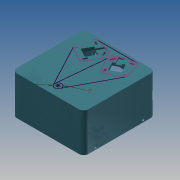
# Autodesk Inventor part: bottom plate box
Saved by Autodesk Inventor 2013 (Build 170138000, 138)
## iProperties
Created: 2017-03-31
Part Number: bottom plate box
Material: Generic
Document SubType Name: Modeling
Designer: employee
Density: 1 g/cm^3
Author: employee
Autodesk Inventor part; units mm, degrees
ref_plane "YZ Plane" through (0, 0, 0) normal (1, 0, 0) x (0, 1, 0)
ref_plane "XZ Plane" through (0, 0, 0) normal (0, 1, 0) x (-1, 0, 0)
sketch "Sketch1" plane through (0, 0, 0) normal (0, 0, 1) x (1, 0, 0)
  circle A0 centre (0, 0) radius 99 construction
  line L0 (0, 103.3586) -> (36.9795, 123.2713) construction
  line L1 (36.9795, 123.2713) -> (56.8922, 86.2918) construction
  line L2 (56.8922, 86.2918) -> (19.9127, 66.3791) construction
  line L3 (19.9127, 66.3791) -> (0, 103.3586) construction
  line L4 (19.9127, 66.3791) -> (0, 0) construction
  line L5 (34.7446, 115.8211) -> (7.4502, 101.1237) construction
  line L6 (7.4502, 101.1237) -> (22.1476, 73.8293) construction
  line L7 (22.1476, 73.8293) -> (49.442, 88.5267) construction
  line L8 (49.442, 88.5267) -> (34.7446, 115.8211) construction
  line L9 (45.2305, 125.1977) -> (56.1863, 84.6519) construction
  line L10 (56.1863, 84.6519) -> (15.6404, 73.696) construction
  line L11 (15.6404, 73.696) -> (4.6846, 114.2419) construction
  line L12 (30.4355, 99.4469) -> (28.9722, 94.6658) construction
  line L13 (0, 103.3586) -> (6.6568, 106.9431)
  line L14 (6.6568, 106.9431) -> (4.6846, 114.2419)
  line L15 (4.6846, 114.2419) -> (45.2305, 125.1977)
  line L16 (45.2305, 125.1977) -> (55.8891, 85.7517)
  line L17 (55.8891, 85.7517) -> (19.9127, 66.3791)
  line L18 (19.9127, 66.3791) -> (0, 103.3586)
  circle A1 centre (49.442, 88.5267) radius 1.75
  circle A2 centre (22.1476, 73.8293) radius 1.75
  circle A3 centre (7.4502, 101.1237) radius 1.75
  circle A4 centre (34.7446, 115.8211) radius 1.75
  line L19 (11.4289, 110.367) -> (41.3556, 118.4535) construction
  line L20 (41.3556, 118.4535) -> (49.442, 88.5267) construction
  line L21 (49.442, 88.5267) -> (19.5153, 80.4403) construction
  line L22 (19.5153, 80.4403) -> (11.4289, 110.367) construction
  circle A5 centre (19.5153, 80.4403) radius 1.75
  circle A6 centre (11.4289, 110.367) radius 1.75
  circle A7 centre (41.3556, 118.4535) radius 1.75
  point P0 (28.4461, 94.8252)
  point P1 (30.4355, 99.4469)
  dimension "d0" = 198
  dimension "d2" = 42
  dimension "d3" = 31
  dimension "d4" = 5.5
  dimension "d5" = 5.5
  dimension "d6" = 5
  dimension "d7" = 3.5
  dimension "d8" = 5.5
  dimension "d9" = 5.5
  constraints: 46 end point, 8 centre point, 8 coincident, 6 equal radius, 6 point on line, 3 collinear, 2 equal length, 2 point on circle, 1 parallel, 1 perpendicular, 1 vertical alignment, 28 other
  measures "d0" diameter of A0
  measures "d2" distance between parallel lines of L1 L3
  measures "d3" distance between parallel lines of L6 L8
  measures "d4" distance from line of L10 L7.end
  measures "d5" distance from line of L9 L7.end
  measures "d6" distance of L12.start L12.end
  measures "d7" diameter of A3
  measures "d8" distance between parallel lines of L22 L11
  measures "d9" distance between parallel lines of L21 L10
extrude "Extrusion1" add sketch "Sketch1" along normal blind 6
fillet "Fillet1" radius 5.5 5 edges at (4.6846, 114.2419, 3) (0, 103.3586, 3) (45.2305, 125.1977, 3) (19.9127, 66.3791, 3) (55.8891, 85.7517, 3)
sketch "Sketch2" plane through (0, 0, 6) normal (0, 0, 1) x (1, 0, 0)
  circle A0 centre (41.3556, 118.4535) radius 1.75 projected
  circle A1 centre (11.4289, 110.367) radius 1.75 projected
  circle A2 centre (19.5153, 80.4403) radius 1.75 projected
  circle A3 centre (34.7446, 115.8211) radius 1.75 projected
  circle A4 centre (7.4502, 101.1237) radius 1.75 projected
  circle A5 centre (22.1476, 73.8293) radius 1.75 projected
  circle A6 centre (49.442, 88.5267) radius 1.75 projected
  arc A7 (12.9463, 109.4952) -> (9.1264, 100.6208) centre (49.442, 88.5267) ccw
  arc A8 (9.9115, 111.2388) -> (5.774, 101.6265) centre (49.442, 88.5267) ccw
  arc A9 (41.8121, 116.7641) -> (35.5743, 114.2803) centre (49.442, 88.5267) ccw
  arc A10 (21.2047, 80.8968) -> (23.6885, 74.659) centre (49.442, 88.5267) ccw
  arc A11 (40.8991, 120.1429) -> (33.9149, 117.362) centre (49.442, 88.5267) ccw
  arc A12 (17.8259, 79.9838) -> (20.6068, 72.9996) centre (49.442, 88.5267) ccw
  point P0 (0, 0)
  constraints: 24 point on circle, 6 centre point, 6 tangent, 4 coincident
extrude "Extrusion2" cut sketch "Sketch2" against normal through all contours A0 A9 A3 A11 | A1 A7 A4 A8 | A2 A10 A5 A12
sketch "Sketch3" plane through (0, 0, 6) normal (0, 0, 1) x (1, 0, 0)
  arc A0 (9.9942, 115.6766) -> (6.1193, 108.9323) centre (11.4289, 110.367) ccw projected
  line L0 (6.1193, 108.9323) -> (6.6568, 106.9431) projected
  line L1 (6.6568, 106.9431) -> (4.8426, 105.9662) projected
  arc A1 (4.8426, 105.9662) -> (2.6076, 98.516) centre (7.4502, 101.1237) ccw projected
  circle A2 centre (49.442, 88.5267) radius 1.75 projected
  arc A3 (6.6599, 113.107) -> (2.1821, 102.704) centre (49.442, 88.5267) ccw
  point P0 (0, 0)
  constraints: 4 point on circle, 1 centre point, 1 coincident, 1 tangent
extrude "Extrusion3" add sketch "Sketch3" against normal up to surface (6 mm away) contours A0 L0 L1 A1 A3
mirror "Mirror1" about plane through (0, 0, 0) normal (1, 0, 0) of "Extrusion1", "Fillet1", "Extrusion2", "Extrusion3"
sketch "Sketch4" plane through (-49.442, 88.5267, 6) normal (0, 0, 1) x (0.9185232, 0.3953672, 0)
  arc A0 (-4.3097, 3.417) -> (-4.3097, -3.417) centre (0, 0) ccw projected
  line L0 (14.9499, -27.7083) -> (-4.3097, -3.417) projected
  arc A1 (14.9499, -27.7083) -> (22.6767, -28.601) centre (19.2596, -24.2913) ccw projected
  line L1 (46.968, -9.3414) -> (22.6767, -28.601) projected
  arc A2 (46.968, -9.3414) -> (49.0146, -5.6629) centre (43.5509, -5.0316) ccw projected
  arc A3 (49.0146, -5.6629) -> (49.0146, 5.6629) centre (0, 0) ccw projected
  arc A4 (49.0146, 5.6629) -> (46.968, 9.3414) centre (43.5509, 5.0316) ccw projected
  line L2 (22.6767, 28.601) -> (46.968, 9.3414) projected
  arc A5 (22.6767, 28.601) -> (14.9499, 27.7083) centre (19.2596, 24.2913) ccw projected
  arc A6 (95.4804, -6.6778) -> (87.9658, -6.4708) centre (90.8273, -39.0955) ccw projected
  arc A7 (94.9832, -10.1423) -> (95.4804, -6.6778) centre (95.2318, -8.41) ccw projected
  arc A8 (94.9832, -10.1423) -> (88.2716, -9.9574) centre (90.8273, -39.0955) ccw projected
  arc A9 (87.9658, -6.4708) -> (88.2716, -9.9574) centre (88.1187, -8.2141) ccw projected
  arc A10 (61.8741, -34.9397) -> (61.6892, -41.6513) centre (90.8273, -39.0955) ccw projected
  arc A11 (58.2026, -41.9571) -> (61.6892, -41.6513) centre (59.9459, -41.8042) ccw projected
  arc A12 (58.4096, -34.4424) -> (58.2026, -41.9571) centre (90.8273, -39.0955) ccw projected
  arc A13 (61.8741, -34.9397) -> (58.4096, -34.4424) centre (60.1418, -34.6911) ccw projected
  arc A14 (63.4972, -2.6049) -> (55.8964, -9.7982) centre (90.8273, -39.0955) ccw projected
  arc A15 (65.5953, -5.4062) -> (63.4972, -2.6049) centre (64.5463, -4.0056) ccw projected
  arc A16 (65.5953, -5.4062) -> (58.5781, -12.0473) centre (90.8273, -39.0955) ccw projected
  arc A17 (55.8964, -9.7982) -> (58.5781, -12.0473) centre (57.2372, -10.9228) ccw projected
  arc A18 (91.3079, -44.5745) -> (96.2715, -39.877) centre (90.8273, -39.0955) ccw projected
  line L3 (96.2715, -39.877) -> (100.676, -9.1914) projected
  arc A19 (100.676, -9.1914) -> (96.0132, -2.9658) centre (95.2318, -8.41) ccw projected
  line L4 (96.0132, -2.9658) -> (65.3277, 1.4387) projected
  arc A20 (65.3277, 1.4387) -> (61.2492, 0.3966) centre (64.5463, -4.0056) ccw projected
  arc A21 (61.2492, 0.3966) -> (53.0232, -7.3884) centre (90.8273, -39.0955) ccw projected
  arc A22 (53.0232, -7.3884) -> (51.7583, -11.4033) centre (57.2372, -10.9228) ccw projected
  line L5 (51.7583, -11.4033) -> (54.4669, -42.2848) projected
  arc A23 (54.4669, -42.2848) -> (60.4265, -47.2832) centre (59.9459, -41.8042) ccw projected
  line L6 (60.4265, -47.2832) -> (91.3079, -44.5745) projected
  circle A24 centre (90.8273, -39.0955) radius 1.75 projected
  circle A25 centre (10.4131, -100.8616) radius 7.5
  line L7 (15.0981, -106.7183) -> (94.263, -43.3904)
  line L8 (2.939, -101.4845) -> (-5.481, -0.4568)
  line L9 (21.4342, 29.3432) -> (97.4063, -3.3581)
  arc A26 (100.676, -9.1914) -> (96.0132, -2.9658) centre (95.2318, -8.41) ccw projected
  line L10 (3.8341, -97.2608) -> (53.0232, -7.3884)
  dimension "d17" = 15
  constraints: 8 end point, 7 point on circle, 7 tangent, 1 centre point, 1 coincident
  measures "d17" diameter of A25
extrude "Extrusion4" add sketch "Sketch4" against normal up to surface (6 mm away) contours A0 L0 A1 L1 A2 A3 A4 L2 A5 L9 A19 L4 A20 A21 A22 L10 A25 L8 | A25 | L10 A22 L5 A23 L6 A18 L7 A25
sketch "Sketch22" plane through (0, 0, 0) normal (0, 0, -1) x (-1, 0, 0)
  arc A0 (-6.6188, -3.5272) -> (6.6188, -3.5272) centre (0, 0) ccw projected
  circle A1 centre (0, 0) radius 4.25
  dimension "d100" = 8.5
  constraints: 1 centre point, 1 coincident
  measures "d100" diameter of A1
extrude "Extrusion22" cut sketch "Sketch22" against normal through all
sketch "Sketch23" plane through (0, 0, 0) normal (0, 0, -1) x (-1, 0, 0)
  arc A0 (-41.3556, 123.9535) -> (-46.6652, 119.8882) centre (-41.3556, 118.4535) ccw projected
  line L0 (-46.6652, 119.8882) -> (-54.7516, 89.9614) projected
  arc A1 (-54.7516, 89.9614) -> (-54.2959, 85.9401) centre (-49.442, 88.5267) ccw projected
  line L1 (-54.2959, 85.9401) -> (-6.6188, -3.5272) projected
  arc A2 (-6.6188, -3.5272) -> (6.6188, -3.5272) centre (0, 0) ccw projected
  line L2 (6.6188, -3.5272) -> (54.2959, 85.9401) projected
  arc A3 (54.2959, 85.9401) -> (54.7516, 89.9614) centre (49.442, 88.5267) ccw projected
  line L3 (46.6652, 119.8882) -> (54.7516, 89.9614) projected
  arc A4 (46.6652, 119.8882) -> (41.3556, 123.9535) centre (41.3556, 118.4535) ccw projected
  line L4 (41.3556, 123.9535) -> (-41.3556, 123.9535) projected
  line L5 (-75, 128.9535) -> (75, 128.9535)
  line L6 (75, 128.9535) -> (75, -21.0465)
  line L7 (75, -21.0465) -> (-75, -21.0465)
  line L8 (-75, -21.0465) -> (-75, 128.9535)
  point P0 (0, 128.9535)
  point P1 (0, 123.9535)
  dimension "d104" = 5
  dimension "d105" = 150
  constraints: 8 end point, 2 midpoint, 2 parallel, 2 perpendicular, 1 horizontal, 1 vertical alignment
  measures "d104" distance between parallel lines of L5 L4
  measures "d105" distance of L5.end L6.end
extrude "Extrusion23" add sketch "Sketch23" against normal up to surface (6 mm away)
fillet "Fillet2" radius 10 4 edges at (-75, 128.9535, 3) (75, 128.9535, 3) (-75, -21.0465, 3) (75, -21.0465, 3)
sketch "Sketch24" plane through (0, 0, 0) normal (0, 0, -1) x (-1, 0, 0)
  arc A0 (-75, -11.0465) -> (-65, -21.0465) centre (-65, -11.0465) ccw projected
  line L0 (65, -21.0465) -> (-65, -21.0465) projected
  arc A1 (65, -21.0465) -> (75, -11.0465) centre (65, -11.0465) ccw projected
  line L1 (75, 118.9535) -> (75, -11.0465) projected
  arc A2 (75, 118.9535) -> (65, 128.9535) centre (65, 118.9535) ccw projected
  line L2 (-65, 128.9535) -> (65, 128.9535) projected
  arc A3 (-65, 128.9535) -> (-75, 118.9535) centre (-65, 118.9535) ccw projected
  line L3 (-75, -11.0465) -> (-75, 118.9535) projected
  arc A4 (70, 118.9535) -> (65, 123.9535) centre (65, 118.9535) ccw
  line L4 (70, 118.9535) -> (70, -11.0465)
  arc A5 (65, -16.0465) -> (70, -11.0465) centre (65, -11.0465) ccw
  line L5 (65, -16.0465) -> (-65, -16.0465)
  arc A6 (-70, -11.0465) -> (-65, -16.0465) centre (-65, -11.0465) ccw
  line L6 (-70, -11.0465) -> (-70, 118.9535)
  arc A7 (-65, 123.9535) -> (-70, 118.9535) centre (-65, 118.9535) ccw
  line L7 (-65, 123.9535) -> (65, 123.9535)
  dimension "d109" = 5
  constraints: 8 end point, 8 point on circle, 4 centre point, 7 other
  measures "d109" distance between parallel lines of L2 L7
extrude "Extrusion24" add sketch "Sketch24" along normal blind 75
sketch "Sketch25" plane through (0, 0, 0) normal (0, 0, -1) x (-1, 0, 0)
  line L0 (-65, -16.0465) -> (65, -16.0465) projected
  circle A0 centre (0, 0) radius 4.25 projected
  line L1 (-12.5, -16.0465) -> (-12.5, 0)
  arc A1 (12.5, 0) -> (-12.5, 0) centre (0, 0) ccw
  line L2 (12.5, 0) -> (12.5, -16.0465)
  dimension "d112" = 12.5
  constraints: 4 end point, 2 perpendicular, 2 point on circle, 2 point on line, 2 tangent, 1 centre point, 1 coincident
  measures "d112" radius of A1
extrude "Extrusion25" add sketch "Sketch25" along normal blind 30
sketch "Sketch26" plane through (0, 0, -30) normal (0, 0, -1) x (-1, 0, 0)
  circle A0 centre (0, 0) radius 4.25 projected
  arc A1 (12.5, 0) -> (-12.5, 0) centre (0, 0) ccw projected
  line L0 (-7.5056, 0) -> (-3.7528, 6.5)
  line L1 (-3.7528, 6.5) -> (3.7528, 6.5)
  line L2 (3.7528, 6.5) -> (7.5056, 0)
  line L3 (7.5056, 0) -> (3.7528, -6.5)
  line L4 (3.7528, -6.5) -> (-3.7528, -6.5)
  line L5 (-3.7528, -6.5) -> (-7.5056, 0)
  dimension "d116" = 13
  constraints: 12 end point, 1 coincident, 1 horizontal, 13 other
  measures "d116" distance between parallel lines of L4 L1
extrude "Extrusion26" cut sketch "Sketch26" against normal blind 8
sketch "Sketch28" plane through (0, 0, 0) normal (0, 0, -1) x (-1, 0, 0)
  circle A0 centre (-49.442, 88.5267) radius 1.75 projected
  arc A1 (-5.774, 101.6265) -> (-9.9115, 111.2388) centre (-49.442, 88.5267) ccw projected
  arc A2 (-9.1264, 100.6208) -> (-5.774, 101.6265) centre (-7.4502, 101.1237) ccw projected
  arc A3 (-9.1264, 100.6208) -> (-12.9463, 109.4952) centre (-49.442, 88.5267) ccw projected
  arc A4 (-9.9115, 111.2388) -> (-12.9463, 109.4952) centre (-11.4289, 110.367) ccw projected
  arc A5 (-33.9149, 117.362) -> (-40.8991, 120.1429) centre (-49.442, 88.5267) ccw projected
  arc A6 (-35.5743, 114.2803) -> (-33.9149, 117.362) centre (-34.7446, 115.8211) ccw projected
  arc A7 (-35.5743, 114.2803) -> (-41.8121, 116.7641) centre (-49.442, 88.5267) ccw projected
  arc A8 (-40.8991, 120.1429) -> (-41.8121, 116.7641) centre (-41.3556, 118.4535) ccw projected
  arc A9 (-23.6885, 74.659) -> (-21.2047, 80.8968) centre (-49.442, 88.5267) ccw projected
  arc A10 (-17.8259, 79.9838) -> (-21.2047, 80.8968) centre (-19.5153, 80.4403) ccw projected
  arc A11 (-20.6068, 72.9996) -> (-17.8259, 79.9838) centre (-49.442, 88.5267) ccw projected
  arc A12 (-23.6885, 74.659) -> (-20.6068, 72.9996) centre (-22.1476, 73.8293) ccw projected
  arc A13 (40.8991, 120.1429) -> (33.9149, 117.362) centre (49.442, 88.5267) ccw projected
  arc A14 (41.8121, 116.7641) -> (40.8991, 120.1429) centre (41.3556, 118.4535) ccw projected
  arc A15 (41.8121, 116.7641) -> (35.5743, 114.2803) centre (49.442, 88.5267) ccw projected
  arc A16 (33.9149, 117.362) -> (35.5743, 114.2803) centre (34.7446, 115.8211) ccw projected
  arc A17 (21.2047, 80.8968) -> (23.6885, 74.659) centre (49.442, 88.5267) ccw projected
  arc A18 (20.6068, 72.9996) -> (23.6885, 74.659) centre (22.1476, 73.8293) ccw projected
  arc A19 (17.8259, 79.9838) -> (20.6068, 72.9996) centre (49.442, 88.5267) ccw projected
  arc A20 (21.2047, 80.8968) -> (17.8259, 79.9838) centre (19.5153, 80.4403) ccw projected
  circle A21 centre (49.442, 88.5267) radius 1.75 projected
  arc A22 (9.9115, 111.2388) -> (5.774, 101.6265) centre (49.442, 88.5267) ccw projected
  arc A23 (12.9463, 109.4952) -> (9.9115, 111.2388) centre (11.4289, 110.367) ccw projected
  arc A24 (12.9463, 109.4952) -> (9.1264, 100.6208) centre (49.442, 88.5267) ccw projected
  arc A25 (5.774, 101.6265) -> (9.1264, 100.6208) centre (7.4502, 101.1237) ccw projected
  arc A26 (-36.1669, 113.1797) -> (-42.1382, 115.5573) centre (-49.442, 88.5267) ccw
  arc A27 (-36.1669, 113.1797) -> (-33.3222, 118.4625) centre (-34.7446, 115.8211) ccw
  arc A28 (-33.3222, 118.4625) -> (-40.573, 121.3496) centre (-49.442, 88.5267) ccw
  arc A29 (-40.573, 121.3496) -> (-42.1382, 115.5573) centre (-41.3556, 118.4535) ccw
  circle A30 centre (-49.442, 88.5267) radius 3
  arc A31 (-24.789, 75.2516) -> (-22.4114, 81.2229) centre (-49.442, 88.5267) ccw
  arc A32 (-24.789, 75.2516) -> (-19.5063, 72.4069) centre (-22.1476, 73.8293) ccw
  arc A33 (-19.5063, 72.4069) -> (-16.6192, 79.6577) centre (-49.442, 88.5267) ccw
  arc A34 (-16.6192, 79.6577) -> (-22.4114, 81.2229) centre (-19.5153, 80.4403) ccw
  arc A35 (-10.3237, 100.2617) -> (-14.0301, 108.8725) centre (-49.442, 88.5267) ccw
  arc A36 (-10.3237, 100.2617) -> (-4.5767, 101.9857) centre (-7.4502, 101.1237) ccw
  arc A37 (-4.5767, 101.9857) -> (-8.8276, 111.8616) centre (-49.442, 88.5267) ccw
  arc A38 (-8.8276, 111.8616) -> (-14.0301, 108.8725) centre (-11.4289, 110.367) ccw
  arc A39 (8.8276, 111.8616) -> (4.5767, 101.9857) centre (49.442, 88.5267) ccw
  arc A40 (14.0301, 108.8725) -> (8.8276, 111.8616) centre (11.4289, 110.367) ccw
  arc A41 (14.0301, 108.8725) -> (10.3237, 100.2617) centre (49.442, 88.5267) ccw
  arc A42 (4.5767, 101.9857) -> (10.3237, 100.2617) centre (7.4502, 101.1237) ccw
  arc A43 (42.1382, 115.5573) -> (36.1669, 113.1797) centre (49.442, 88.5267) ccw
  arc A44 (42.1382, 115.5573) -> (40.573, 121.3496) centre (41.3556, 118.4535) ccw
  arc A45 (40.573, 121.3496) -> (33.3222, 118.4625) centre (49.442, 88.5267) ccw
  arc A46 (33.3222, 118.4625) -> (36.1669, 113.1797) centre (34.7446, 115.8211) ccw
  arc A47 (16.6192, 79.6577) -> (19.5063, 72.4069) centre (49.442, 88.5267) ccw
  arc A48 (19.5063, 72.4069) -> (24.789, 75.2516) centre (22.1476, 73.8293) ccw
  arc A49 (22.4114, 81.2229) -> (24.789, 75.2516) centre (49.442, 88.5267) ccw
  arc A50 (22.4114, 81.2229) -> (16.6192, 79.6577) centre (19.5153, 80.4403) ccw
  circle A51 centre (49.442, 88.5267) radius 3
  dimension "d124" = 3
  constraints: 48 point on circle, 26 centre point, 7 equal radius, 18 other
  measures "d124" radius of A29
extrude "Extrusion28" cut sketch "Sketch28" against normal blind 3
sketch "Sketch31" plane through (-65, 123.9535, 0) normal (0, -1, 0) x (1, 0, 0)
  circle A0 centre (18.9, -18.5) radius 1.75 construction
  circle A1 centre (113.85, -48.125) radius 1.75 construction
  circle A2 centre (113.85, -27.875) radius 1.75 construction
  circle A3 centre (18.9, -57.5) radius 1.75 construction
  line L0 (117.6, -15) -> (12.4, -15) construction
  line L1 (12.4, -15) -> (12.4, -61) construction
  line L2 (12.4, -61) -> (117.6, -61) construction
  line L3 (117.6, -61) -> (117.6, -15) construction
  line L4 (122.6, -66) -> (7.4, -66)
  line L5 (7.4, -66) -> (7.4, -10)
  line L6 (7.4, -10) -> (122.6, -10)
  line L7 (122.6, -10) -> (122.6, -66)
  point P0 (65, 0)
  dimension "d135" = 5
  constraints: 8 end point, 3 other
  measures "d135" distance between parallel lines of L1 L5
extrude "Extrusion31" add sketch "Sketch31" along normal blind 5.6
chamfer "Chamfer2" distance 5.6 angle 45 1 edges at (0, 123.9535, -10)
sketch "Sketch32" plane through (-65, 128.9535, 6) normal (0, 1, 0) x (1, 0, 0)
  line L0 (122.6, 16) -> (7.4, 16) projected
  circle A0 centre (18.9, 24.5) radius 1.75 projected
  circle A1 centre (113.85, 54.125) radius 1.75 projected
  circle A2 centre (113.85, 33.875) radius 1.75 projected
  circle A3 centre (18.9, 63.5) radius 1.75 projected
  line L1 (117.6, 21) -> (12.4, 21) projected
  line L2 (12.4, 21) -> (12.4, 67) projected
  line L3 (12.4, 67) -> (117.6, 67) projected
  line L4 (117.6, 67) -> (117.6, 21) projected
  line L5 (11.9, 20.5) -> (118.1, 20.5)
  line L6 (118.1, 20.5) -> (118.1, 67.5)
  line L7 (118.1, 67.5) -> (11.9, 67.5)
  line L8 (11.9, 67.5) -> (11.9, 20.5)
  line L9 (7.4, 72) -> (122.6, 72) projected
  line L10 (122.6, 72) -> (122.6, 16) projected
  line L11 (7.4, 16) -> (7.4, 72) projected
  point P0 (65, 6)
  dimension "d141" = 0.5
  constraints: 8 end point, 3 other
  measures "d141" distance between parallel lines of L5 L1
ref_plane "Work Plane4" through (-52.6, 120.3535, -61) normal (0, -1, 0) x (1, 0, 0)
extrude "Extrusion32" cut sketch "Sketch32" against normal up to surface (8.6 mm away) contours A0 | A1 | A2 | A3 | L1 L2 L3 L4 | L8 L7 L6 L5
chamfer "Chamfer3" distance 8.6 angle 45 1 edges at (0, 128.9535, -61.5)
sketch "Sketch33" plane through (-53.1, 120.3535, -14.5) normal (0, 1, 0) x (1, 0, 0)
  circle A0 centre (7, 4) radius 1.75 projected
  circle A1 centre (101.95, 33.625) radius 1.75 projected
  circle A2 centre (101.95, 13.375) radius 1.75 projected
  circle A3 centre (7, 43) radius 1.75 projected
  line L0 (98.2, 29.25) -> (105.7, 29.25) projected
  line L1 (105.7, 29.25) -> (105.7, 46.5) projected
  line L2 (105.7, 46.5) -> (0.5, 46.5) projected
  line L3 (0.5, 46.5) -> (0.5, 0.5) projected
  line L4 (0.5, 0.5) -> (105.7, 0.5) projected
  line L5 (105.7, 0.5) -> (105.7, 17.75) projected
  line L6 (105.7, 17.75) -> (98.2, 17.75) projected
  line L7 (98.2, 17.75) -> (98.2, 4) projected
  line L8 (98.2, 4) -> (40.7, 4) projected
  line L9 (40.7, 4) -> (40.7, 38) projected
  line L10 (40.7, 38) -> (98.2, 38) projected
  line L11 (98.2, 38) -> (98.2, 29.25) projected
  circle A4 centre (21.5, 23.5) radius 16 projected
  point P0 (53.1, -14.5)
extrude "Extrusion33" cut sketch "Sketch33" against normal up to next contours A0 | A1 | A2 | A3
sketch "Sketch34" plane through (-53.1, 120.3535, -14.5) normal (0, 1, 0) x (1, 0, 0)
  circle A0 centre (7, 43) radius 1.75 projected
  line L0 (106.2, 47) -> (0, 47) projected
  line L1 (10, 47) -> (96.2, 47)
  line L2 (96.2, 47) -> (96.2, 0)
  line L3 (96.2, 0) -> (10, 0)
  line L4 (10, 0) -> (10, 47)
  line L5 (106.2, 0) -> (0, 0) projected
  point P0 (53.1, -14.5)
  point P1 (53.1, 47)
  point P2 (53.1, 47)
  dimension "d149" = 3
  constraints: 8 end point, 2 midpoint, 2 parallel, 2 point on line, 1 coincident, 1 horizontal, 1 perpendicular
  measures "d149" distance from line of L4 A0.centre
extrude "Extrusion34" cut sketch "Sketch34" against normal up to next contours L2 L3 L4 L0
sketch "Sketch35" plane through (53.1, 120.3535, -14.5) normal (-1, 0, 0) x (0, 0, 1)
  line L0 (-55.6, 8.6) -> (0, 8.6) projected
  line L1 (-17.95, 4.1) -> (-17.95, 5.4) construction
  line L2 (-17.95, 5.4) -> (-29.05, 5.4) construction
  line L3 (-29.05, 5.4) -> (-29.05, 4.1) construction
  line L4 (-29.05, 4.1) -> (-17.95, 4.1) construction
  line L5 (-46.5, 0) -> (-0.5, 0) projected
  line L6 (-46.5, 0) -> (-46.5, 1.6) projected
  line L7 (-29.25, 1.6) -> (-46.5, 1.6) projected
  line L8 (-29.25, 1.6) -> (-29.25, 5.6) construction
  line L9 (-17.75, 5.6) -> (-29.25, 5.6) construction
  line L10 (-17.75, 1.6) -> (-17.75, 5.6) construction
  line L11 (-0.5, 1.6) -> (-17.75, 1.6) projected
  line L12 (-0.5, 0) -> (-0.5, 1.6) projected
  line L13 (-35.55, 8.6) -> (-30.05, 3.1)
  line L14 (-30.05, 3.1) -> (-16.95, 3.1)
  line L15 (-16.95, 3.1) -> (-11.45, 8.6)
  point P0 (14.5, -120.3535)
  point P1 (-23.5, 3.1)
  point P2 (-23.5, 4.1)
  dimension "d152" = 1
  dimension "d153" = 1
  constraints: 6 end point, 2 midpoint, 2 perpendicular, 2 point on line, 1 parallel, 1 vertical alignment
  measures "d152" distance between parallel lines of L4 L14
  measures "d153" horizontal distance of L13.end L3.end
sketch "Sketch36" plane through (57.6, 118.3535, -66) normal (1, 0, 0) x (0, 0, -1)
  line L0 (-61.6, 5.6) -> (0, 5.6) projected
  line L1 (-56, 0) -> (-61.6, 5.6) projected
  line L2 (0, 0) -> (-56, 0) projected
  line L3 (0, 5.6) -> (0, 0) projected
  point P0 (-66, -118.3535)
extrude "Extrusion35" add sketch "Sketch36" along normal up to next
extrude "Extrusion36" cut sketch "Sketch35" against normal through all
sketch "Sketch37" plane through (0, 0, 0) normal (0, 0, -1) x (-1, 0, 0)
  arc A0 (12.5, 0) -> (-12.5, 0) centre (0, 0) ccw projected
  line L0 (-65, -16.0465) -> (-12.5, -16.0465) projected
  line L1 (-44.44, 66.9135) -> (44.44, 66.9135) construction
  line L2 (44.44, 66.9135) -> (44.44, 23.9535) construction
  line L3 (44.44, 23.9535) -> (-44.44, 23.9535) construction
  line L4 (-44.44, 23.9535) -> (-44.44, 66.9135) construction
  circle A1 centre (-44.44, 66.9135) radius 1.5
  circle A2 centre (-44.44, 66.9135) radius 4
  circle A3 centre (-44.44, 23.9535) radius 1.5
  circle A4 centre (-44.44, 23.9535) radius 4
  circle A5 centre (44.44, 23.9535) radius 1.5
  circle A6 centre (44.44, 23.9535) radius 4
  circle A7 centre (44.44, 66.9135) radius 1.5
  circle A8 centre (44.44, 66.9135) radius 4
  point P0 (0, 23.9535)
  dimension "d158" = 88.88
  dimension "d160" = 42.96
  dimension "d161" = 3
  dimension "d162" = 8
  dimension "d163" = 40
  constraints: 8 centre point, 8 coincident, 8 end point, 6 equal radius, 2 parallel, 1 horizontal, 1 midpoint, 1 perpendicular, 1 vertical alignment
  measures "d158" distance of L1.start L1.end
  measures "d160" distance of L3.end L1.start
  measures "d161" diameter of A3
  measures "d162" diameter of A4
  measures "d163" distance between parallel lines of L3 L0
extrude "Extrusion37" add sketch "Sketch37" along normal blind 10
sketch "Sketch38" plane through (0, 0, 6) normal (0, 0, 1) x (1, 0, 0)
  arc A0 (40.8991, 120.1429) -> (33.9149, 117.362) centre (49.442, 88.5267) ccw projected
  arc A1 (20.6068, 72.9996) -> (23.6885, 74.659) centre (22.1476, 73.8293) ccw projected
  arc A2 (5.774, 101.6265) -> (9.1264, 100.6208) centre (7.4502, 101.1237) ccw projected
  line L0 (7.4502, 101.1237) -> (22.1476, 73.8293)
  line L1 (22.1476, 73.8293) -> (49.442, 88.5267)
  line L2 (49.442, 88.5267) -> (34.7446, 115.8211)
  line L3 (34.7446, 115.8211) -> (7.4502, 101.1237)
  line L4 (32.7128, 109.0483) -> (42.6692, 90.5585)
  line L5 (42.6692, 90.5585) -> (24.1794, 80.6021)
  line L6 (24.1794, 80.6021) -> (14.2231, 99.0919)
  line L7 (14.2231, 99.0919) -> (32.7128, 109.0483)
  line L8 (19.0656, 101.6995) -> (27.8703, 106.4406)
  line L9 (27.8703, 106.4406) -> (20.7586, 119.6476)
  line L10 (20.7586, 119.6476) -> (11.9539, 114.9065)
  line L11 (11.9539, 114.9065) -> (19.0656, 101.6995)
  point P0 (23.4679, 104.0701)
  dimension "d166" = 10
  dimension "d169" = 5
  dimension "d170" = 36
  constraints: 24 end point, 6 parallel, 3 perpendicular, 2 midpoint, 2 point on line, 1 coincident, 3 other
  measures "d166" distance between parallel lines of L9 L11
  measures "d169" distance between parallel lines of L1 L5
  measures "d170" distance between parallel lines of L10 L5
extrude "Extrusion38" cut sketch "Sketch38" against normal blind 3 contours L11 L10 L9 L3 | L3 L9 L7 L11 | L7 L4 L5 L6
sketch "Sketch39" plane through (0, 0, 3) normal (0, 0, 1) x (1, 0, 0)
  line L0 (14.2231, 99.0919) -> (19.0656, 101.6995) projected
  line L1 (14.2231, 99.0919) -> (32.7128, 109.0483)
  line L2 (32.7128, 109.0483) -> (42.6692, 90.5585)
  line L3 (42.6692, 90.5585) -> (24.1794, 80.6021)
  line L4 (24.1794, 80.6021) -> (14.2231, 99.0919)
  point P0 (0, 0)
  constraints: 8 end point, 2 parallel, 1 collinear, 1 perpendicular
extrude "Extrusion39" cut sketch "Sketch39" against normal through all
mirror "Mirror3" about plane through (0, 0, 0) normal (1, 0, 0) of "Extrusion38", "Extrusion39"
sketch "Sketch40" plane through (-65, 128.9535, 6) normal (0, 1, 0) x (1, 0, 0)
  line L0 (130, 56.05) -> (130, 81) projected
  line L1 (0, 81) -> (130, 81) projected
  circle A0 centre (127, 66) radius 6
  circle A1 centre (127, 66) radius 5.25
  point P0 (65, 6)
  dimension "d175" = 12
  dimension "d177" = 15
  dimension "d178" = 3
  dimension "d179" = 10.5
  constraints: 2 centre point, 1 coincident
  measures "d175" diameter of A0
  measures "d177" distance from line of L1 A0.centre
  measures "d178" distance from line of L0 A0.centre
  measures "d179" diameter of A1
extrude "Extrusion40" cut sketch "Sketch40" against normal blind 4 contours A1 L0 | L0 A1
sketch "Sketch41" plane through (62, 124.9535, -60) normal (0, 1, 0) x (1, 0, 0)
  circle A0 centre (0, 0) radius 5.25 projected
  circle A1 centre (0, 0) radius 4
  point P0 (-62, -60)
  dimension "d182" = 8
  constraints: 1 centre point, 1 coincident
  measures "d182" diameter of A1
extrude "Extrusion41" cut sketch "Sketch41" against normal up to surface (6.6 mm away) contours A1
sketch "Sketch42" plane through (-65, 118.3535, 0) normal (0, -1, 0) x (1, 0, 0)
  circle A0 centre (127, -60) radius 4 projected
  line L0 (135, -10) -> (135, -66) projected
  line L1 (7.4, -66) -> (135, -66) projected
  arc A1 (127, -52) -> (119, -60) centre (127, -60) ccw
  line L2 (119, -60) -> (119, -66)
  line L3 (7.4, -10) -> (7.4, -66) projected
  line L4 (127, -52) -> (135, -52)
  point P0 (65, 0)
  point P1 (135, -60)
  constraints: 4 end point, 3 point on line, 3 tangent, 2 perpendicular, 2 point on circle, 1 centre point, 1 coincident
extrude "Extrusion42" cut sketch "Sketch42" against normal blind 3.1
chamfer "Chamfer4" distance 2 angle 45 3 edges at (56.3431, 118.3535, -54.3431) (66, 118.3535, -52) (54, 118.3535, -63)
fillet "Fillet3" radius 2 6 edges at (66, 120.3535, -52) (54, 120.3535, -63) (56.3431, 120.3535, -54.3431) (52, 118.3535, -63) (66, 118.3535, -50) (54.9289, 118.3535, -52.9289)
sketch "Sketch43" plane through (75, -11.0465, 6) normal (1, 0, 0) x (0, 0, -1)
  line L0 (81, 130) -> (81, 0) projected
  circle A0 centre (76, 115) radius 1.75
  circle A1 centre (76, 15) radius 1.75
  line L1 (76, 115) -> (76, 15) construction
  point P0 (6, 11.0465)
  point P1 (76, 65)
  point P2 (81, 65)
  dimension "d193" = 3.5
  dimension "d195" = 100
  dimension "d196" = 5
  constraints: 2 centre point, 2 end point, 2 midpoint, 1 equal radius, 1 horizontal alignment, 1 parallel
  measures "d193" diameter of A1
  measures "d195" distance of L1.start L1.end
  measures "d196" distance between parallel lines of L1 L0
extrude "Extrusion43" cut sketch "Sketch43" against normal through all
sketch "Sketch44" plane through (75, -11.0465, 6) normal (1, 0, 0) x (0, 0, -1)
  circle A0 centre (76, 115) radius 1.75 projected
  circle A1 centre (76, 15) radius 1.75 projected
  circle A2 centre (76, 15) radius 3
  circle A3 centre (76, 115) radius 3
  point P0 (6, 11.0465)
  dimension "d199" = 6
  constraints: 2 centre point, 2 coincident, 1 equal radius
  measures "d199" diameter of A3
extrude "Extrusion44" cut sketch "Sketch44" against normal blind 3
sketch "Sketch45" plane through (-75, -11.0465, 6) normal (-1, 0, 0) x (0, 0, 1)
  circle A0 centre (-76, 115) radius 1.75 projected
  circle A1 centre (-76, 15) radius 1.75 projected
  circle A2 centre (-76, 115) radius 3 projected
  circle A3 centre (-76, 15) radius 3 projected
  point P0 (-6, 11.0465)
extrude "Extrusion45" cut sketch "Sketch45" against normal blind 3
ref_plane "Work Plane2" through (-65, 53.9535, 6) normal (0, -1, 0) x (1, 0, 0)
ref_plane "Work Plane3" through (0, -11.0465, 6) normal (-1, 0, 0) x (0, 0, 1)
sketch "Sketch27" plane through (-75, -11.0465, 6) normal (-1, 0, 0) x (0, 0, 1)
  line L0 (-81, 0) -> (-81, 130) projected
  line L1 (5, 130) -> (5, 0) construction
  line L2 (5, 0) -> (-81, 0) construction
  line L3 (-81, 0) -> (-81, 130) construction
  line L4 (-81, 130) -> (5, 130) construction
  point P0 (-6, 11.0465)
  constraints: 1 coincident, 1 collinear, 2 other
body "Solid1"
